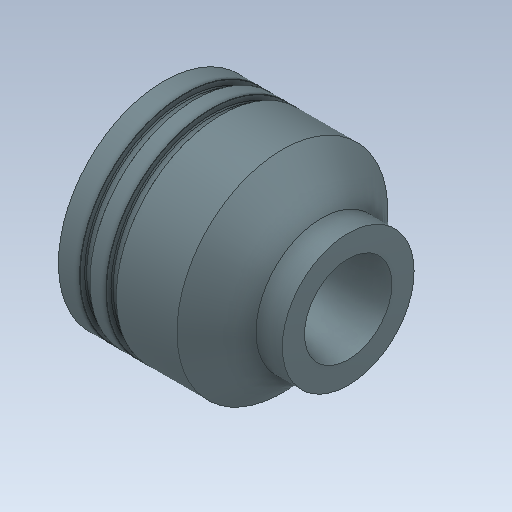
# Autodesk Inventor part: ODSY-0003-102
Saved by Autodesk Inventor 2021 (Build 250183000, 183)
## iProperties
Company: ERPL
Created: 2021-10-20
Material: Generic
Document SubType Name: Modeling
Designer: ALEX CLAY
Density: 2.26947 g/cm^3
Appearance: Lead
Mass: 1043.26 g
Surface Area: 482.002 cm^2
Volume: 459.694 cm^3
Project: ODYSSEY
Description: NOZZLE INSERT
Part Number: ODSY-0003-102
Author: ALEX CLAY
Revision Number: 00
Autodesk Inventor part; units mm, degrees
ref_plane "YZ Plane" through (0, 0, 0) normal (1, 0, 0) x (0, 1, 0)
derived "Rao Nozzle.ipt"
sketch "Sketch1" plane through (0, 0, 0) normal (0, 0, 1) x (1, 0, 0)
  arc A0 (-10.3341, 13.9464) -> (0, 9.525) centre (0, 23.8125) ccw
  arc A1 (0, 9.525) -> (1.2445, 9.7444) centre (0, 13.1635) ccw
  line L0 (-7.4701, 9.525) -> (9.7854, 9.525) construction
  line L1 (-10.3341, 13.9464) -> (-37.5801, 42.4849)
  arc A2 (46.7269, 21.0845) -> (1.2445, 9.7444) centre (77.9324, -200.954) ccw
  line L2 (1.2445, 9.7444) -> (30.761, 20.4876) construction
  line L3 (46.7269, 21.0845) -> (89.89, 27.1507) construction
  line L4 (46.7269, 21.0845) -> (95.911, 21.0845) construction
  line L5 (-42.1731, 50.8) -> (46.7269, 50.8)
  line L6 (46.7269, 50.8) -> (46.7269, 21.0845)
  line L7 (-72.1769, 0) -> (123.9257, 0)
  arc A3 (-37.5801, 42.4849) -> (-42.1731, 44.45) centre (-42.1731, 38.1) ccw
  line L8 (-42.1731, 44.45) -> (-42.1731, 50.8)
  line L9 (46.7269, 31.75) -> (34.0269, 31.75)
  line L10 (34.0269, 31.75) -> (14.9769, 50.8)
  point P0 (0, 0)
revolve "Revolution1" add sketch "Sketch1" angle 360 about axis through (-10, 0, 0) along (1, 0, 0) contours L1 A3 L8 L5 L10 L9 L6 A2 A1 A0
sketch "Sketch2" plane through (0, 0, 0) normal (0, 1, 0) x (-1, 0, 0)
  line L0 (31.848, -50.8) -> (27.0982, -50.8)
  line L1 (27.0982, -50.8) -> (27.0982, -47.9806)
  line L2 (27.0982, -47.9806) -> (31.848, -47.9806)
  line L3 (31.848, -47.9806) -> (31.848, -50.8)
  line L4 (19.148, -47.9806) -> (14.3982, -47.9806)
  line L5 (14.3982, -47.9806) -> (14.3982, -50.8)
  line L6 (14.3982, -50.8) -> (19.148, -50.8)
  line L7 (19.148, -50.8) -> (19.148, -47.9806)
  line L8 (29.4731, -50.8) -> (29.4731, -97.9888) construction
  line L9 (16.7731, -50.8) -> (16.7731, -101.7212) construction
  line L10 (42.1731, 50.8) -> (42.1731, -50.8) projected
  line L11 (57.1258, 0) -> (-9.521, 0) projected
  point P0 (0, 0)
  dimension "d2" = 4.7498
  dimension "d3" = 4.7498
  dimension "d4" = 2.8194
  dimension "d5" = 12.7
  dimension "d6" = 12.7
  constraints: 20 end point, 4 parallel, 2 collinear, 2 horizontal, 2 midpoint, 2 perpendicular, 2 vertical, 1 point on line
  measures "d2" distance of L0.start L0.end
  measures "d3" distance of L5.end L6.end
  measures "d4" distance of L4.end L5.end
  measures "d5" distance between parallel lines of L9 L8
  measures "d6" distance between parallel lines of L8 L10
revolve "Revolution2" cut sketch "Sketch2" angle 360 about axis through (-10, 0, 0) along (1, 0, 0)
fillet "Fillet1" radius 0.508 4 edges at (-14.3982, 0, 47.9806) (-27.0982, 0, 47.9806) (-19.148, 0, 47.9806) (-31.848, 0, 47.9806)
fillet "Fillet2" radius 0.127 4 edges at (-31.848, -50.8, 0) (-27.0982, -50.8, 0) (-19.148, -50.8, 0) (-14.3982, -50.8, 0)
ref_plane "Work Plane1" through (-29.4731, 0, 0) normal (-1, 0, 0) x (0, 0, 1)
ref_plane "Work Plane2" through (-16.7731, 0, 0) normal (1, 0, 0) x (0, 0, -1)
body "Solid1"
